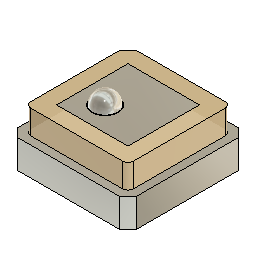
GPSモジュール (Autodesk Fusion 360 design; units mm, degrees)
Autodesk Fusion 360 part; units mm, degrees
sketch "スケッチ1" plane through (0, 0, 0) normal (0, 0, 1) x (1, 0, 0)
  line L0 (8.9, -10.4) -> (-8.9, -10.4)
  line L1 (-10.4, -8.9) -> (-10.4, 8.9)
  line L2 (-8.9, 10.4) -> (8.9, 10.4)
  line L3 (10.4, 8.9) -> (10.4, -8.9)
  line L4 (10.4, -10.4) -> (-10.4, 10.4) construction
  line L5 (-10.4, -10.4) -> (10.4, 10.4) construction
  line L6 (-10.4, 8.9) -> (-8.9, 10.4)
  line L7 (-8.9, -10.4) -> (-10.4, -8.9)
  line L8 (10.4, -8.9) -> (8.9, -10.4)
  line L9 (8.9, 10.4) -> (10.4, 8.9)
  dimension "d1" = 20.8
  dimension "d2" = 20.8
  dimension "d3" = 1.5
  dimension "d5" = 360
  constraint horizontal L0
  constraint perpendicular L0 L1
  constraint parallel L0 L2
  constraint parallel L1 L3
  constraint coincident L4 origin
  constraint coincident L5 origin
  constraint perpendicular L4 L6
  measures "d1" distance of L4.end L5.end
  measures "d2" distance of L5.start L4.end
  measures "d3" distance of L4.end L1.end
extrude "押し出し1" add sketch "スケッチ1" along normal blind 5
sketch "スケッチ2" plane through (0, 0, 5) normal (0, 0, 1) x (-1, 0, 0)
  line L0 (-8.9, -10.4) -> (8.9, -10.4)
  line L1 (8.9, -10.4) -> (10.4, -8.9)
  line L2 (10.4, -8.9) -> (10.4, 8.9)
  line L3 (10.4, 8.9) -> (8.9, 10.4)
  line L4 (8.9, 10.4) -> (-8.9, 10.4)
  line L5 (-8.9, 10.4) -> (-10.4, 8.9)
  line L6 (-10.4, 8.9) -> (-10.4, -8.9)
  line L7 (-10.4, -8.9) -> (-8.9, -10.4)
  line L8 (7.5, -9) -> (-8, -9)
  line L9 (-9, -8) -> (-9, 8)
  line L10 (-8, 9) -> (8, 9)
  line L11 (9, 8) -> (9, -7.5)
  line L12 (9, -7.5) -> (7.5, -9)
  arc A0 (-9, -8) -> (-8, -9) centre (-8, -8) ccw
  arc A1 (-8, 9) -> (-9, 8) centre (-8, 8) ccw
  arc A2 (9, 8) -> (8, 9) centre (8, 8) ccw
  point P0 (-9, -9)
  point P1 (-9, 9)
  point P2 (9, 9)
  dimension "d8" = 18
  dimension "d9" = 18
  dimension "d11" = 1
  constraint horizontal L8
  constraint perpendicular L8 L9
  constraint parallel L8 L10
  constraint parallel L9 L11
  constraint coincident P0 L8
  constraint coincident P0 L9
  constraint tangent L8 A0
  constraint tangent L9 A0
  constraint coincident P1 L9
  constraint coincident P1 L10
  constraint tangent L9 A1
  constraint tangent L10 A1
  constraint equal A0 A1
  constraint coincident P2 L10
  constraint coincident P2 L11
  constraint tangent L10 A2
  constraint tangent L11 A2
  constraint equal A0 A2
  measures "d8" distance of P1 P2
  measures "d9" distance of P0 P1
  measures "d11" radius of A0
extrude "押し出し2" add sketch "スケッチ2" along normal blind 4.2 contours L8 L9 L10 L11 L12 A0 A1 A2 picked at (3, 3.5)
sketch "スケッチ3" plane through (0, 0, 9.2) normal (0, 0, 1) x (-1, 0, 0)
  line L0 (9, -7.5) -> (9, 8)
  arc A0 (9, 8) -> (8, 9) centre (8, 8) ccw
  line L1 (8, 9) -> (-8, 9)
  arc A1 (-8, 9) -> (-9, 8) centre (-8, 8) ccw
  line L2 (-9, 8) -> (-9, -8)
  arc A2 (-9, -8) -> (-8, -9) centre (-8, -8) ccw
  line L3 (-8, -9) -> (7.5, -9)
  line L4 (7.5, -9) -> (9, -7.5)
  line L5 (-6.25, 6.25) -> (6.25, 6.25)
  line L6 (6.25, 6.25) -> (6.25, -6.25)
  line L7 (6.25, -6.25) -> (-6.25, -6.25)
  line L8 (-6.25, -6.25) -> (-6.25, 6.25)
  line L9 (-6.25, 6.25) -> (6.25, -6.25) construction
  line L10 (6.25, 6.25) -> (-6.25, -6.25) construction
  dimension "d14" = 12.5
  dimension "d15" = 12.5
  constraint horizontal L5
  constraint perpendicular L5 L6
  constraint parallel L5 L7
  constraint parallel L6 L8
  constraint coincident L9 origin
  constraint coincident L10 origin
  measures "d14" distance of L6.end L7.end
  measures "d15" distance of L5.end L6.end
extrude "押し出し3" cut sketch "スケッチ3" against normal blind 0.0001 contours L5 L6 L7 L8 picked at (-2.083333, 2.083333)
sphere "球プリミティブ1" add diameter 4.4 placed x (-1, 0, 0) y (0, -1, 0) z (0, 0, 1) at (-2, -2, 9.1999)
sketch "スケッチ5" plane through (0, 0, 9.1999) normal (0, 0, 1) x (-1, 0, 0)
  circle A0 centre (2, 2) radius 2.2
  line L0 (-6.25, -6.25) -> (6.25, -6.25)
  line L1 (6.25, -6.25) -> (6.25, 6.25)
  line L2 (6.25, 6.25) -> (-6.25, 6.25)
  line L3 (-6.25, 6.25) -> (-6.25, -6.25)
  circle A1 centre (2, 2) radius 2.2
  circle A2 centre (2, 2) radius 2.3
  dimension "d19" = 4.4
  dimension "d20" = 0.1
  constraint concentric A0 A1
  measures "d19" diameter of A1
extrude "押し出し4" cut sketch "スケッチ5" against normal blind 0.00001 contours A2 picked at (4.249913, 1.776437)
